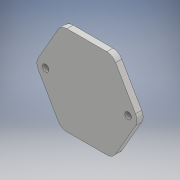
# Autodesk Inventor part: Battery cover hex
Saved by Autodesk Inventor 2017 (Build 210142000, 142)
## iProperties
Created: 2017-05-16
Part Number: Battery cover hex
Material: Generic
Document SubType Name: Modeling
Designer: yella
Density: 1 g/cm^3
Appearance: Default
Author: yella
Autodesk Inventor part; units mm, degrees
ref_plane "YZ Plane" through (0, 0, 0) normal (1, 0, 0) x (0, 1, 0)
ref_plane "XZ Plane" through (0, 0, 0) normal (0, 1, 0) x (-1, 0, 0)
ref_plane "XY Plane" through (0, 0, 0) normal (0, 0, 1) x (1, 0, 0)
sketch "Sketch1" plane through (0, 0, 0) normal (0, 1, 0) x (-1, 0, 0)
  line L0 (23.5566, -2.5) -> (13.9434, -19.1506)
  line L1 (9.6132, -21.6506) -> (-9.6132, -21.6506)
  line L2 (-13.9434, -19.1506) -> (-23.5566, -2.5)
  line L3 (-23.5566, 2.5) -> (-13.9434, 19.1506)
  line L4 (-9.6132, 21.6506) -> (9.6132, 21.6506)
  line L5 (13.9434, 19.1506) -> (23.5566, 2.5)
  line L6 (0, 0) -> (20, 0)
  line L7 (0, 0) -> (-20, 0)
  circle A0 centre (20, 0) radius 1.6
  circle A1 centre (-20, 0) radius 1.6
  arc A2 (13.9434, 19.1506) -> (9.6132, 21.6506) centre (9.6132, 16.6506) ccw
  arc A3 (23.5566, -2.5) -> (23.5566, 2.5) centre (19.2265, 0) ccw
  arc A4 (9.6132, -21.6506) -> (13.9434, -19.1506) centre (9.6132, -16.6506) ccw
  arc A5 (-13.9434, -19.1506) -> (-9.6132, -21.6506) centre (-9.6132, -16.6506) ccw
  arc A6 (-23.5566, 2.5) -> (-23.5566, -2.5) centre (-19.2265, 0) ccw
  arc A7 (-9.6132, 21.6506) -> (-13.9434, 19.1506) centre (-9.6132, 16.6506) ccw
  point P0 (25, 0)
  point P1 (12.5, -21.6506)
  point P2 (-12.5, -21.6506)
  point P3 (-25, 0)
  point P4 (-12.5, 21.6506)
  point P5 (12.5, 21.6506)
  dimension "d0" = 50
  dimension "d1" = 20
  dimension "d2" = 20
  dimension "d3" = 3.2
  dimension "d4" = 3.2
  dimension "d5" = 5
  constraints: 16 end point, 12 point on circle, 12 point on line, 12 tangent, 8 centre point, 5 equal radius, 3 coincident, 2 horizontal, 13 other
  measures "d0" distance of point (-25, 0) point (25, 0)
  measures "d1" distance of L6.start L6.end
  measures "d2" distance of L6.start L7.end
  measures "d3" diameter of A0
  measures "d4" diameter of A1
  measures "d5" radius of A2
extrude "Extrusion1" add sketch "Sketch1" along normal blind 3
body "Solid1"
